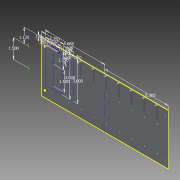
# Autodesk Inventor part: BoardOutline
Saved by Autodesk Inventor 2013 (Build 170138000, 138)
## iProperties
Created: 2012-08-24
Part Number: BoardOutline
Material: Generic
Document SubType Name: Modeling
Designer: henry
Density: 1 g/cm^3
Author: henry
Autodesk Inventor part; units mm, degrees
ref_plane "YZ Plane" through (0, 0, 0) normal (1, 0, 0) x (0, 1, 0)
ref_plane "XZ Plane" through (0, 0, 0) normal (0, 1, 0) x (-1, 0, 0)
ref_plane "XY Plane" through (0, 0, 0) normal (0, 0, 1) x (1, 0, 0)
sketch "Sketch1" plane through (0, 0, 0) normal (0, 0, 1) x (1, 0, 0)
  line L0 (0, 0) -> (-254, 0)
  line L1 (-254, 0) -> (-254, 101.6)
  line L2 (-254, 101.6) -> (0, 101.6)
  line L3 (0, 101.6) -> (0, 0)
  line L4 (0, 101.6) -> (-254, 0)
  dimension "d0" = 254
  dimension "d1" = 101.6
  constraints: 10 end point, 2 parallel, 1 horizontal, 1 perpendicular
  measures "d0" distance of L1.end L2.end
  measures "d1" distance of L2.end L0.start
extrude "Extrusion1" add sketch "Sketch1" along normal blind 1.5875
sketch "Sketch2" plane through (0, 0, 1.5875) normal (0, 0, 1) x (1, 0, 0)
  line L0 (-254, 101.6) -> (0, 101.6) projected
  line L1 (-254, 0) -> (-254, 101.6) projected
  line L2 (0, 101.6) -> (0, 0) projected
  line L3 (-254, 12.7) -> (2.7117, 12.7)
  line L4 (-254, 88.9) -> (0, 88.9)
  line L5 (-247.65, 88.9) -> (-247.65, 12.7)
  line L6 (-6.35, 88.9) -> (-6.35, 12.7)
  dimension "d4" = 76.2
  dimension "d5" = 12.7
  dimension "d6" = 241.3
  dimension "d29" = 6.35
  constraints: 8 end point, 7 point on line, 4 coincident, 3 perpendicular, 1 parallel
  measures "d4" distance between parallel lines of L3 L4
  measures "d5" distance between parallel lines of L0 L4
  measures "d6" distance between parallel lines of L6 L5
  measures "d29" distance between parallel lines of L5 L1
hole "Hole1" at (-247.65, 88.9, 1.5875) at (-247.65, 12.7, 1.5875) at (-6.35, 12.7, 1.5875) at (-6.35, 88.9, 1.5875) direction (0, 0, -1) diameter 3.175 end through all
sketch "Sketch4" plane through (0, 0, 1.5875) normal (0, 0, 1) x (1, 0, 0)
  line L0 (-254, 101.6) -> (0, 101.6) projected
  line L1 (-254, 0) -> (-254, 101.6) projected
  line L2 (0, 0) -> (-254, 0) projected
  line L3 (0, 101.6) -> (0, 0) projected
  point P0 (-281.0349, 34.925)
  point P1 (-280.9828, 73.025)
  dimension "d36" = 28.575
  dimension "d37" = 38.1
  measures "d36" distance from line of point (-280.983, 73.025) L0
  measures "d37" distance of point (-281.035, 34.925) point (-280.983, 73.025)
sketch "Sketch3" plane through (0, 0, 1.5875) normal (0, 0, 1) x (1, 0, 0)
  line L0 (0, 0) -> (-254, 0) projected
  line L1 (0, 101.6) -> (0, 0) projected
  line L2 (-246.0625, 98.425) -> (-214.3125, 98.425) construction
  line L3 (-214.3125, 98.425) -> (-214.3125, 22.225) construction
  line L4 (-214.3125, 22.225) -> (-246.0625, 22.225) construction
  line L5 (-246.0625, 22.225) -> (-246.0625, 98.425) construction
  line L6 (-230.1875, 22.225) -> (-230.1875, 98.425) construction
  line L7 (-218.1875, 95.25) -> (-242.1875, 91.25) construction
  line L8 (-127, 101.6) -> (-127, -0.7428) construction
  line L9 (-254, 101.6) -> (0, 101.6) construction
  line L10 (-218.1875, 95.25) -> (-242.1875, 95.25)
  line L11 (-242.1875, 95.25) -> (-242.1875, 91.25)
  line L12 (-242.1875, 91.25) -> (-218.1875, 91.25)
  line L13 (-218.1875, 91.25) -> (-218.1875, 95.25)
  circle A0 centre (-247.65, 12.7) radius 1.5875 projected
  circle A1 centre (-247.65, 88.9) radius 1.5875 projected
  line L14 (-254, 101.6) -> (0, 101.6) projected
  line L15 (-254, 0) -> (-254, 101.6) projected
  line L16 (0, 0) -> (-254, 0) projected
  line L17 (0, 101.6) -> (0, 0) projected
  point P0 (-230.1875, 66.675)
  point P1 (-230.1875, 28.575)
  point P2 (-230.1875, 93.25)
  dimension "d19" = 31.75
  dimension "d20" = 15.875
  dimension "d30" = 76.2
  dimension "d31" = 31.75
  dimension "d32" = 38.1
  dimension "d33" = 127
  dimension "d34" = 119.0625
  dimension "d35" = 3.175
  dimension "d50" = 4
  dimension "d51" = 24
  dimension "d52" = 6.35
  constraints: 22 end point, 4 midpoint, 4 parallel, 4 perpendicular, 3 point on line, 2 horizontal
  measures "d19" distance between parallel lines of L3 L5
  measures "d20" distance between parallel lines of L5 L6
  measures "d30" distance between parallel lines of L2 L4
  measures "d31" distance from line of L2 point (-230.188, 66.675)
  measures "d32" distance of point (-230.188, 66.675) point (-230.188, 28.575)
  measures "d33" distance between parallel lines of L1 L8
  measures "d34" distance between parallel lines of L5 L8
  measures "d35" distance between parallel lines of L9 L2
  measures "d50" distance of L10.end L7.end
  measures "d51" distance of L7.start L10.end
  measures "d52" distance between parallel lines of L9 L10
hole "Hole2" at (-230.1875, 28.575, 1.5875) at (-230.1875, 66.675, 1.5875) direction (0, 0, -1) diameter 3.175 end through all
extrude "Extrusion3" add sketch "Sketch3" along normal blind 4 contours L13 L12 L11 L10
sketch "Sketch6" plane through (0, 0, 1.5875) normal (0, 0, 1) x (1, 0, 0)
  line L0 (-254, 101.6) -> (0, 101.6) projected
  line L1 (-254, 0) -> (-254, 101.6) projected
  line L2 (-209.55, 98.425) -> (-190.5, 98.425) construction
  line L3 (-190.5, 98.425) -> (-190.5, 22.225) construction
  line L4 (-190.5, 22.225) -> (-209.55, 22.225) construction
  line L5 (-209.55, 22.225) -> (-209.55, 98.425) construction
  line L6 (-200.025, 98.425) -> (-200.025, 22.225) construction
  line L7 (-198.025, 76.327) -> (-198.025, 100.33)
  line L8 (-198.025, 100.33) -> (-202.025, 100.33)
  line L9 (-202.025, 100.33) -> (-202.025, 76.327)
  line L10 (-202.025, 76.327) -> (-198.025, 76.327)
  line L11 (-198.025, 76.327) -> (-202.025, 100.33) construction
  line L12 (-198.025, 100.33) -> (-202.025, 76.327) construction
  point P0 (-200.025, 88.3285)
  dimension "d58" = 19.05
  dimension "d61" = 76.2
  dimension "d62" = 44.45
  dimension "d63" = 3.175
  dimension "d64" = 4
  dimension "d65" = 24.003
  dimension "d66" = 1.27
  constraints: 22 end point, 5 parallel, 4 midpoint, 2 perpendicular, 1 horizontal, 1 point on line
  measures "d58" distance of L2.start L2.end
  measures "d61" distance of L2.end L3.end
  measures "d62" distance between parallel lines of L1 L5
  measures "d63" distance between parallel lines of L0 L2
  measures "d64" distance of L7.end L8.end
  measures "d65" distance between parallel lines of L8 L10
  measures "d66" distance between parallel lines of L8 L0
extrude "Extrusion4" add sketch "Sketch6" along normal blind 4
sketch "Sketch7" plane through (0, 0, 1.5875) normal (0, 0, 1) x (1, 0, 0)
  line L0 (-202.025, 100.33) -> (-198.025, 100.33) projected
  line L1 (-242.1875, 95.25) -> (-218.1875, 95.25) projected
  line L2 (0, 101.6) -> (0, 0) projected
  line L3 (-200.025, 100.33) -> (-200.025, 19.4799) construction
  point P0 (-200.025, 66.675)
  point P1 (-200.025, 15.875)
  dimension "d69" = 28.575
  dimension "d70" = 50.8
  constraints: 2 end point, 2 point on line, 1 midpoint, 1 parallel
  measures "d69" distance from line of L1 point (-200.025, 66.675)
  measures "d70" distance of point (-200.025, 66.675) point (-200.025, 15.875)
hole "Hole3" at (-200.025, 15.875, 1.5875) at (-200.025, 66.675, 1.5875) direction (0, 0, -1) diameter 3.175 end through all
pattern_linear "Rectangular Pattern3" count 8 spacing 25.4 along (1, 0, 0) of "Extrusion4", "Hole3"
body "Solid1"
